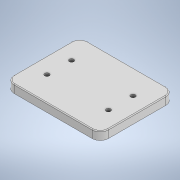
# Autodesk Inventor part: stand
Saved by Autodesk Inventor 2020 (Build 240168000, 168)
## iProperties
Created: 2020-08-08
Part Number: stand
Material: Generic
Document SubType Name: Modeling
Designer: benny
Density: 1 g/cm^3
Appearance: Default
Author: benny
Autodesk Inventor part; units mm, degrees
ref_plane "YZ Plane" through (0, 0, 0) normal (1, 0, 0) x (0, 1, 0)
ref_plane "XZ Plane" through (0, 0, 0) normal (0, 1, 0) x (-1, 0, 0)
ref_plane "XY Plane" through (0, 0, 0) normal (0, 0, 1) x (1, 0, 0)
sketch "Sketch1" plane through (0, 0, 0) normal (0, 1, 0) x (-1, 0, 0)
  line L0 (115, 90) -> (-115, 90)
  line L1 (-115, 90) -> (-115, -90)
  line L2 (-115, -90) -> (115, -90)
  line L3 (115, -90) -> (115, 90)
  line L4 (115, 90) -> (-115, -90) construction
  line L5 (-115, 90) -> (115, -90) construction
  point P0 (0, 0)
  dimension "d0" = 230
  dimension "d1" = 180
  constraints: 12 end point, 2 midpoint, 2 parallel, 1 horizontal, 1 perpendicular
  measures "d0" distance of L2.end L1.end
  measures "d1" distance of L1.end L0.end
extrude "Extrusion1" add sketch "Sketch1" along normal blind 20
fillet "Fillet1" radius 2 4 edges at (0, 20, 90) (115, 20, 0) (0, 20, -90) (-115, 20, 0)
fillet "Fillet2" radius 20 8 edges at (-114.4142, 19.4142, 89.4142) (-115, 9, 90) (114.4142, 19.4142, 89.4142) (115, 9, 90) (-115, 9, -90) (-114.4142, 19.4142, -89.4142) (114.4142, 19.4142, -89.4142) (115, 9, -90)
sketch "Sketch2" plane through (0, 20, 0) normal (0, 1, 0) x (1, 0, 0)
  line L0 (75, 30) -> (0, 0)
  circle A0 centre (75, 30) radius 5.5
  dimension "d6" = 11
  constraints: 2 end point, 1 centre point, 1 coincident
  measures "d6" diameter of A0
extrude "Extrusion2" cut sketch "Sketch2" against normal blind 20
sketch "Sketch3" plane through (0, 0, 0) normal (0, -1, 0) x (1, 0, 0)
  circle A0 centre (75, -30) radius 5.5 projected
  circle A1 centre (75, -30) radius 9
  point P0 (0, 0)
  dimension "d9" = 18
  constraints: 1 centre point, 1 coincident
  measures "d9" diameter of A1
extrude "Extrusion3" cut sketch "Sketch3" against normal blind 11 contours A0 | A1
mirror "Mirror1" about plane through (0, 0, 0) normal (0, 0, 1) of "Extrusion2", "Extrusion3"
mirror "Mirror2" about plane through (0, 0, 0) normal (1, 0, 0) of "Extrusion2", "Extrusion3", "Mirror1"
body "Solid1"
